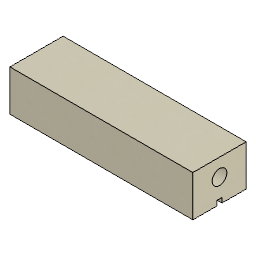
F1 In Schools Model Block Jig (Autodesk Fusion 360 archive; units mm, degrees)
design "F1 In Schools Model Block Polyurethane"
Autodesk Fusion 360 part; units mm, degrees
sketch "Sketch1" plane through (0, 0, 0) normal (1, 0, 0) x (0, 1, 0)
  line L0 (-32.5, 25) -> (32.5, 25)
  line L1 (32.5, 25) -> (32.5, -25)
  line L2 (-32.5, -25) -> (-32.5, 25)
  line L3 (-3, -19) -> (3, -19)
  line L4 (3, -19) -> (3, -25)
  line L5 (-3, -25) -> (-3, -19)
  line L6 (32.5, -25) -> (3, -25)
  line L7 (-3, -25) -> (-32.5, -25)
  circle A0 centre (0, 4) radius 9
  dimension "d1" = 65
  dimension "d2" = 50
  dimension "d3" = 6
  dimension "d4" = 6
  dimension "d7" = 18
  constraint horizontal L0
  constraint vertical L1
  constraint horizontal L6
  constraint vertical L2
  constraint horizontal L3
  constraint vertical L4
  constraint vertical L5
  constraint collinear L6 L7
  measures "d1" distance of L0.start L0.end
  measures "d2" distance of L0.start L2.start
  measures "d3" distance of L3.start L3.end
  measures "d4" distance of L3.start L5.start
  measures "d7" diameter of A0
extrude "Extrude1" add sketch "Sketch1" against normal blind 223 makes body 1
delete_face "DeleteFace1" 1 faces at (-74.3333, 8.9553, 3.1039) on bodies 1
extrude "Extrude2" cut sketch "Sketch1" against normal blind 52 contours A0 bodies 1
ref_plane "WorkPlane1" through (-55, 0, 0) normal (1, 0, 0) x (0, 1, 0)
sketch "Sketch2" plane through (-55, 0, 0) normal (1, 0, 0) x (0, 1, 0)
  circle A0 centre (0, 4) radius 0.05
  dimension "d13" = 0.1
  measures "d13" diameter of A0
delete_face "DeleteFace2" 1 faces at (-34.6667, 8.9553, 3.1039) on bodies 1
extrude "Extrude3" cut sketch "Sketch1" against normal blind 52.01 contours A0 bodies 1
ref_plane "WorkPlane2" through (-52, 0, 0) normal (1, 0, 0) x (0, 1, 0)
split "Split1" by plane through (-52, 0, 0) normal (1, 0, 0) bodies 1 makes body 2 at (-17.3333, -10.8333, 25)
loft "Loft1" cut section 1 face at (-52.01, -4.4271, 5.6952) section 2 point at (-55, 0, 4) on bodies 1 bodies 1
combine "Combine1" operation add target body 2 tool bodies 1
move_body "Move1" bodies 2 to x (1, 0, 0) y (0, 1, 0) z (0, 0, 1) at (111.5, 0, 0)
